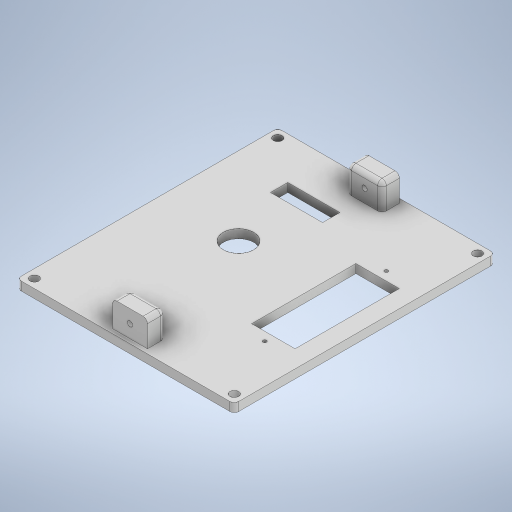
# Autodesk Inventor part: top
Saved by Autodesk Inventor 2024 (Build 280153000, 153)
## iProperties
Created: 2026-03-15
Part Number: top
Material: Generic
Document SubType Name: Modeling
Designer: HP
Density: 1 g/cm^3
Appearance: Default
Author: HP
Autodesk Inventor part; units mm, degrees
ref_plane "YZ Plane" through (0, 0, 0) normal (1, 0, 0) x (0, 1, 0)
ref_plane "XZ Plane" through (0, 0, 0) normal (0, 1, 0) x (-1, 0, 0)
ref_plane "XY Plane" through (0, 0, 0) normal (0, 0, 1) x (1, 0, 0)
sketch "Sketch1" plane through (0, 0, 0) normal (0, 1, 0) x (-1, 0, 0)
  line L0 (0, 0) -> (0, 150)
  line L1 (0, 150) -> (125, 150)
  line L2 (125, 150) -> (125, -150)
  line L3 (125, -150) -> (-125, -150)
  line L4 (-125, -150) -> (-125, 150)
  line L5 (-125, 150) -> (0, 150)
  line L6 (125, 150) -> (125, 140)
  line L7 (125, 140) -> (115, 140)
  circle A0 centre (115, 140) radius 5
  line L8 (125, 0) -> (-125, 0)
  line L9 (0, 150) -> (0, -150)
  circle A1 centre (115, -140) radius 5
  circle A2 centre (-115, 140) radius 5
  circle A3 centre (-115, -140) radius 5
  dimension "d0" = 150
  dimension "d1" = 125
  dimension "d2" = 300
  dimension "d3" = 250
  dimension "d4" = 10
  dimension "d5" = 10
  dimension "d6" = 10
  constraints: 20 end point, 6 perpendicular, 4 centre point, 3 midpoint, 3 symmetric about line, 2 point on line, 1 coincident, 1 vertical, 3 other
  measures "d0" distance of L0.start L0.end
  measures "d1" distance of L0.end L1.end
  measures "d2" distance of L1.end L2.end
  measures "d3" distance of L2.end L3.end
  measures "d4" distance of L1.end L6.end
  measures "d5" distance of L6.end L7.end
  measures "d6" diameter of A0
extrude "Extrusion1" add sketch "Sketch1" along normal blind 10
fillet "Fillet1" radius 5 4 edges at (-125, 5, 150) (-125, 5, -150) (125, 5, -150) (125, 5, 150)
sketch "Sketch2" plane through (0, 10, 0) normal (0, 1, 0) x (1, 0, 0)
  line L0 (-120, -150) -> (120, -150) projected
  line L1 (-117.475, -150) -> (-117.475, -145)
  line L2 (125, -145) -> (125, 145) projected
  line L3 (-117.475, -145) -> (125, -145)
  line L4 (0, 0) -> (0, -145)
  line L5 (0, -145) -> (-20, -145)
  line L6 (-20, -145) -> (-20, -125)
  line L7 (-20, -125) -> (20, -125)
  line L8 (20, -125) -> (20, -145)
  line L9 (-125, 145) -> (-125, -145) projected
  line L10 (-125, 0) -> (125, 0)
  line L11 (-117.475, 145) -> (125, 145)
  line L12 (-20, 145) -> (-20, 125)
  line L13 (-20, 125) -> (20, 125)
  line L14 (20, 125) -> (20, 145)
  dimension "d10" = 5
  dimension "d11" = 20
  dimension "d12" = 20
  dimension "d13" = 40
  constraints: 24 end point, 6 point on line, 5 symmetric about line, 4 perpendicular, 2 midpoint, 1 vertical
  measures "d10" distance of L1.start L1.end
  measures "d11" distance of L4.end L5.end
  measures "d12" distance of L5.end L6.end
  measures "d13" distance of L6.end L7.end
extrude "Extrusion2" add sketch "Sketch2" along normal blind 30 contours L14 L13 L12 L11 | L3 L4 L7 L8 | L3 L6 L7 L4
fillet "Fillet2" radius 5 10 edges at (-20, 40, -135) (20, 40, -135) (-20, 40, 135) (20, 40, 135) (20, 25, 125) (20, 25, -125) (-20, 25, -125) (-20, 25, 125) (0, 40, 125) (0, 40, -125)
sketch "Sketch3" plane through (20, 10, -145) normal (0, 0, -1) x (-1, 0, 0)
  line L0 (40, 0) -> (40, 25) projected
  line L1 (40, 0) -> (20, 0)
  line L2 (140, 0) -> (-100, 0) projected
  line L3 (20, 0) -> (20, 15)
  circle A0 centre (20, 15) radius 3
  point P0 (20, -10)
  dimension "d17" = 20
  dimension "d18" = 15
  dimension "d19" = 6
  constraints: 4 end point, 1 centre point, 1 coincident, 1 midpoint, 1 perpendicular
  measures "d17" distance of L0.start L1.end
  measures "d18" distance of L1.end L3.end
  measures "d19" diameter of A0
hole "Hole1" at (0, 25, -145) direction (0, 0, 1) diameter 6 end through all
sketch "Sketch4" plane through (0, 10, 0) normal (0, 1, 0) x (1, 0, 0)
  line L0 (125, -145) -> (125, 145) projected
  line L1 (125, 0) -> (105, 0)
  line L2 (105, 0) -> (105, -60)
  line L3 (105, -60) -> (55, -60)
  line L4 (55, -60) -> (55, 60)
  line L5 (55, 60) -> (105, 60)
  line L6 (105, 60) -> (105, 0)
  line L7 (105, 0) -> (80, 0)
  line L8 (80, 0) -> (80, -70)
  circle A0 centre (80, -70) radius 2
  circle A1 centre (80, 70) radius 2
  point P0 (0, 0)
  dimension "d27" = 20
  dimension "d28" = 60
  dimension "d29" = 50
  dimension "d30" = 120
  dimension "d31" = 25
  dimension "d32" = 70
  dimension "d33" = 4
  constraints: 16 end point, 6 perpendicular, 2 centre point, 2 point on line, 1 coincident, 1 horizontal, 1 midpoint, 1 symmetric about line, 1 other
  measures "d27" distance of L1.start L1.end
  measures "d28" distance of L1.end L2.end
  measures "d29" distance of L2.end L3.end
  measures "d30" distance of L3.end L4.end
  measures "d31" distance of L1.end L7.end
  measures "d32" distance of L7.end L8.end
  measures "d33" diameter of A0
extrude "Extrusion3" cut sketch "Sketch4" against normal blind 30
sketch "Sketch5" plane through (0, 0, 0) normal (0, -1, 0) x (1, 0, 0)
  line L0 (-125, -145) -> (-125, 145) projected
  line L1 (-125, 0) -> (-35, 0)
  line L2 (-35, 0) -> (-35, -120.65)
  line L3 (-35, -120.65) -> (-35, 114.35)
  line L4 (-35, -120.65) -> (-35, -84.15)
  line L5 (-35, -101.6) -> (-65, -101.6)
  line L6 (-65, -101.6) -> (-5, -101.6)
  line L7 (-65, -101.6) -> (-65, -81.6)
  line L8 (-65, -81.6) -> (-5, -81.6)
  line L9 (-5, -81.6) -> (-5, -101.6)
  line L10 (-35, -81.6) -> (-35, -14.85)
  circle A0 centre (-35, -14.85) radius 17.5
  line L11 (-35, 2.6) -> (-35, 118.15)
  circle A1 centre (-35, 118.15) radius 7.5
  point P0 (0, 0)
  dimension "d36" = 90
  dimension "d37" = 235
  dimension "d38" = 36.5
  dimension "d39" = 30
  dimension "d40" = 60
  dimension "d41" = 20
  dimension "d42" = 66.75
  dimension "d43" = 35
  dimension "d44" = 115.55
  dimension "d45" = 15
  constraints: 22 end point, 4 point on line, 2 centre point, 2 coincident, 2 horizontal, 2 perpendicular, 2 vertical, 1 midpoint
  measures "d36" distance of L1.start L1.end
  measures "d37" distance of L2.end L3.end
  measures "d38" distance of L4.end L2.end
  measures "d39" distance of L5.start L5.end
  measures "d40" distance of L5.end L6.end
  measures "d41" distance of L5.end L7.end
  measures "d42" distance of L10.start L10.end
  measures "d43" diameter of A0
  measures "d44" distance of L11.start L11.end
  measures "d45" diameter of A1
extrude "Extrusion4" cut sketch "Sketch5" against normal blind 10
body "Solid1"
